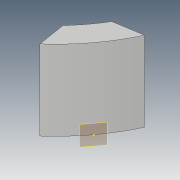
# Autodesk Inventor part: landingGear2
Saved by Autodesk Inventor 2018 (Build 220112000, 112)
## iProperties
Created: 2020-02-26
Part Number: landingGear2
Material: Generic
Document SubType Name: Modeling
Designer: anirudh.bali
Density: 1 g/cm^3
Appearance: Default
Author: anirudh.bali
Autodesk Inventor part; units mm, degrees
ref_plane "YZ Plane" through (0, 0, 0) normal (1, 0, 0) x (0, 1, 0)
ref_plane "XZ Plane" through (0, 0, 0) normal (0, 1, 0) x (-1, 0, 0)
ref_plane "XY Plane" through (0, 0, 0) normal (0, 0, 1) x (1, 0, 0)
sketch "Sketch1" plane through (0, 0, 0) normal (0, 1, 0) x (-1, 0, 0)
  line L0 (-159.8042, 152.4) -> (-154.8717, 121.8603)
  arc A0 (-154.8717, 121.8603) -> (-178.2507, 90.8267) centre (-25.4, 0) ccw
  line L1 (-178.2507, 90.8267) -> (-209.614, 85.7638)
  arc A1 (-154.8717, 121.8603) -> (-178.2507, 90.8267) centre (-25.4, 0) ccw
  arc A2 (-159.8042, 152.4) -> (-209.614, 85.7638) centre (-25.4, 0) ccw
  circle A3 centre (-166.4316, 128.5066) radius 1.75
  circle A4 centre (-187.8284, 100.1043) radius 1.75
  point P0 (0, 0)
  constraints: 6 point on circle, 5 centre point, 4 coincident, 4 end point
extrude "Extrusion1" add sketch "Sketch1" along normal blind 88.9
sketch "Sketch2" plane through (0, 0, 0) normal (0, -1, 0) x (1, 0, 0)
  arc A0 (209.614, 85.7638) -> (159.8042, 152.4) centre (25.4, 0) ccw projected
  line L0 (0, 0) -> (209.614, 85.7638)
  line L1 (209.614, 85.7638) -> (209.614, 85.7638)
  line L2 (209.614, 85.7638) -> (209.614, 85.7638)
  line L3 (209.614, 85.7638) -> (209.614, 85.7638)
  line L4 (0, 0) -> (159.8042, 152.4)
  line L5 (209.614, 85.7638) -> (178.2507, 90.8267) projected
  line L6 (159.8042, 152.4) -> (209.614, 85.7638)
  line L7 (0, 0) -> (184.7091, 119.0819)
  line L8 (188.3344, 121.4192) -> (184.7091, 119.0819)
  constraints: 16 end point, 1 collinear, 1 midpoint, 1 point on circle, 1 point on line
ref_plane "Work Plane1" through (188.3344, 0, 121.4192) normal (0.8018427, 0, 0.5975352) x (0, 1, 0)
sketch "Sketch5" plane through (0, 0, 0) normal (0, -1, 0) x (1, 0, 0)
  circle A0 centre (187.8284, 100.1043) radius 2.1971
  circle A1 centre (166.4316, 128.5066) radius 2.1971
  point P0 (0, 0)
  dimension "d9" = 4.3942
  dimension "d10" = 4.3942
  constraints: 2 centre point, 2 coincident
  measures "d9" diameter of A0
  measures "d10" diameter of A1
extrude "Extrusion3" cut sketch "Sketch5" against normal blind 4.8006
sketch "Sketch6" plane through (0, 88.9, 0) normal (0, 1, 0) x (1, 0, 0)
  circle A0 centre (166.4316, -128.5066) radius 1.75 projected
  circle A1 centre (166.4316, -128.5066) radius 1.75
  circle A2 centre (187.8284, -100.1043) radius 2.1971 projected
  circle A3 centre (187.8284, -100.1043) radius 1.75
  point P0 (0, 0)
  constraints: 2 centre point, 2 coincident
extrude "Extrusion4" add sketch "Sketch6" against normal blind 84.0994 contours A0 | A3
body "Solid1"
